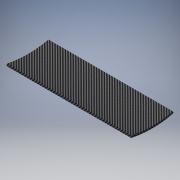
# Autodesk Inventor part: element_2
Saved by Autodesk Inventor 2018.1 (Build 221171000, 171)
## iProperties
Created: 2017-10-18
Part Number: element_2
Material: CFRP
Document SubType Name: Modeling
Designer: kuwano
Density: 1.43 g/cm^3
Appearance: カーボンファイバー
Mass: 45.1089 g
Surface Area: 224.286 cm^2
Volume: 31.5447 cm^3
Author: kuwano
Autodesk Inventor part; units mm, degrees
ref_plane "YZ Plane" through (0, 0, 0) normal (1, 0, 0) x (0, 1, 0)
ref_plane "XZ Plane" through (0, 0, 0) normal (0, 1, 0) x (-1, 0, 0)
ref_plane "XY Plane" through (0, 0, 0) normal (0, 0, 1) x (1, 0, 0)
sketch "スケッチ1" plane through (0, 0, 0) normal (1, 0, 0) x (0, 1, 0)
  arc A0 (6.2855, 30) -> (6.2855, -30) centre (141.6068, 0) ccw
  arc A1 (3.3566, 30.6493) -> (3.3566, -30.6493) centre (141.6068, 0) ccw
  line L0 (6.2855, 30) -> (3.3566, 30.6493)
  line L1 (6.2855, -30) -> (3.3566, -30.6493)
  line L2 (0, -42.909) -> (0, 42.909) projected
  point P0 (0, 0)
  point P1 (0, 0)
  dimension "d0" = 3
  dimension "d1" = 60
  dimension "d2" = 25
  constraints: 5 point on circle, 4 end point, 4 line through centre, 2 centre point, 1 coincident, 1 concentric, 1 tangent
  measures "d0" distance of L0.start L0.end
  measures "d1" distance of L1.start L0.start
  measures "d2" angle of L1 L0
extrude "押し出し1" add sketch "スケッチ1" along normal blind 180
sketch "スケッチ2" plane through (0, 0, 0) normal (-1, 0, 0) x (0, 0, 1)
  arc A0 (-30.6493, 3.3566) -> (30.6493, 3.3566) centre (0, 141.6068) ccw projected
  line L0 (-30.6493, 3.3566) -> (-6.3173, -2.0376)
  line L1 (-30.6493, 3.3566) -> (-30, 6.2855) projected
  line L2 (-30.5411, 3.8448) -> (-18.9336, 1.2715)
  point P0 (0, 0)
  dimension "d5" = 0.5
  constraints: 4 end point, 1 parallel, 1 point on circle, 1 point on line, 1 tangent
  measures "d5" distance from line of L0.start L2
extrude "押し出し2" cut sketch "スケッチ2" against normal through all
sketch "スケッチ3" plane through (0, 0, 0) normal (-1, 0, 0) x (0, 0, 1)
  line L0 (-5, 0.0883) -> (5, 0.0883)
  arc A0 (-18.9336, 1.2715) -> (30.6493, 3.3566) centre (0, 141.6068) ccw projected
  point P0 (0, 0)
  dimension "d9" = 10
  constraints: 2 end point, 2 point on circle, 1 horizontal
  measures "d9" distance of L0.start L0.end
extrude "押し出し3" cut sketch "スケッチ3" against normal through all
